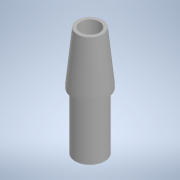
# Autodesk Inventor part: Barrel to Tip Stopper
Saved by Autodesk Inventor 2020 (Build 240168000, 168)
## iProperties
Created: 2020-03-16
Part Number: Barrel to Tip Stopper
Material: Generic
Document SubType Name: Modeling
Designer: Daniel
Density: 1 g/cm^3
Appearance: Light Gray
Author: Daniel
Autodesk Inventor part; units mm, degrees
ref_plane "YZ Plane" through (0, 0, 0) normal (1, 0, 0) x (0, 1, 0)
ref_plane "XZ Plane" through (0, 0, 0) normal (0, 1, 0) x (-1, 0, 0)
ref_plane "XY Plane" through (0, 0, 0) normal (0, 0, 1) x (1, 0, 0)
sketch "Sketch1" plane through (0, 0, 0) normal (0, 0, 1) x (1, 0, 0)
  line L0 (0, 0) -> (0, -4.2026)
  line L1 (2.1336, 8.4974) -> (3.302, 8.4974)
  line L2 (3.302, 8.4974) -> (3.302, -4.2026)
  line L3 (3.302, -4.2026) -> (2.1336, -4.2026)
  line L4 (2.1336, -4.2026) -> (2.1336, 8.4974)
  line L5 (2.1336, 8.4974) -> (3.937, 8.4974)
  line L6 (3.937, 8.4974) -> (3.937, 9.4118)
  line L7 (3.937, 9.4118) -> (2.1336, 9.4118)
  line L8 (2.1336, 9.4118) -> (2.1336, 8.4974)
  line L9 (2.8483, 20.3338) -> (2.1336, 20.3338)
  line L10 (2.1336, 20.3338) -> (2.1336, 16.0248)
  line L11 (2.8483, 20.3338) -> (3.937, 9.4118)
  line L12 (2.1336, 16.0248) -> (2.1336, 9.3134)
  dimension "d0" = 3.302
  dimension "d1" = 2.1336
  dimension "d2" = 12.7
  dimension "d3" = 3.937
  dimension "d4" = 0.9144
  dimension "d6" = 10.922
  constraints: 26 end point, 4 parallel, 2 horizontal, 2 perpendicular, 1 point on line, 1 vertical
  measures "d0" distance between parallel lines of L0 L2
  measures "d1" distance between parallel lines of L0 L4
  measures "d2" distance of L1.end L2.end
  measures "d3" distance between parallel lines of L6 L0
  measures "d4" distance of L5.end L6.end
  measures "d6" distance from line of L9 L6.end
revolve "Revolution1" add sketch "Sketch1" angle 360 about axis through (0, 0, 0) along (0, -1, 0)
body "Solid1"
